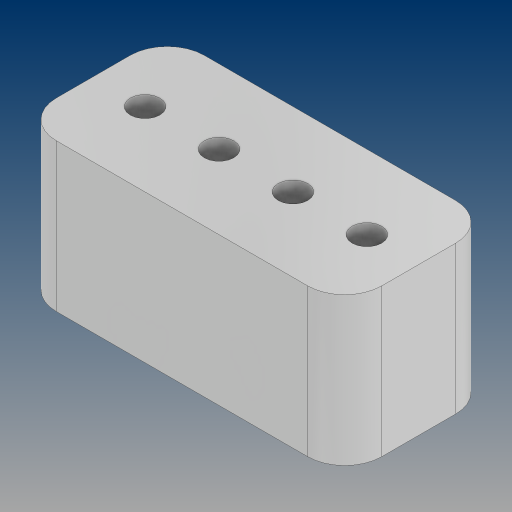
# Autodesk Inventor part: ELEV_020_BILLET1(Shit)
Saved by Autodesk Inventor 2024.3 (Build 283343000, 343)
## iProperties
Created: 2024-11-28
Part Number: ELEV_020_BILLET1(Shit)
Material: Aluminum 6061
Document SubType Name: Modeling
Designer: Kenji
Mass: 91.6842 g
Surface Area: 83.689 cm^2
Volume: 33.9571 cm^3
Density: 2.7 g/cm^3
Appearance: Aluminum - Polished
Author: Kenji
Autodesk Inventor part; units mm, degrees
ref_plane "YZ Plane" through (0, 0, 0) normal (1, 0, 0) x (0, 1, 0)
ref_plane "XZ Plane" through (0, 0, 0) normal (0, 1, 0) x (-1, 0, 0)
ref_plane "XY Plane" through (0, 0, 0) normal (0, 0, 1) x (1, 0, 0)
sketch "Sketch1" plane through (0, 0, 0) normal (0, 1, 0) x (-1, 0, 0)
  line L0 (0, 0) -> (55.88, 0)
  line L1 (55.88, 0) -> (55.88, -25.4)
  line L2 (55.88, -25.4) -> (0, -25.4)
  line L3 (0, -25.4) -> (0, 0)
  circle A0 centre (46.99, -12.7) radius 2.54
  circle A1 centre (34.29, -12.7) radius 2.54
  circle A2 centre (21.59, -12.7) radius 2.54
  circle A3 centre (8.89, -12.7) radius 2.54
  line L4 (55.88, -12.7) -> (0, -12.7) construction
  dimension "d0" = 25.4
  dimension "d1" = 55.88
  dimension "d2" = 5.08
  dimension "d3" = 12.7
  dimension "d4" = 12.7
  dimension "d5" = 12.7
  dimension "d6" = 12.7
  dimension "d7" = 8.89
  constraints: 10 end point, 4 centre point, 4 point on line, 3 equal radius, 2 midpoint, 2 parallel, 2 perpendicular, 1 horizontal
  measures "d0" distance between parallel lines of L2 L0
  measures "d1" distance between parallel lines of L3 L1
  measures "d2" diameter of A3
  measures "d3" distance between parallel lines of L0 L4
  measures "d4" distance of A2.centre A3.centre
  measures "d5" distance of A1.centre A2.centre
  measures "d6" distance of A0.centre A1.centre
  measures "d7" distance from line of L1 A0.centre
extrude "Extrusion1" add sketch "Sketch1" along normal blind 25.4
fillet "Fillet1" radius 6.35 4 edges at (-55.88, 12.7, 0) (-55.88, 12.7, -25.4) (0, 12.7, -25.4) (0, 12.7, 0)
body "Solid1"
